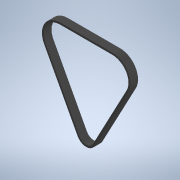
# Autodesk Inventor part: Belt_A
Saved by Autodesk Inventor 2020 (Build 240168000, 168)
## iProperties
Created: 2020-03-07
Part Number: Belt_A
Material: Rubber
Document SubType Name: Modeling
Designer: 10300812
Density: 0.93 g/cm^3
Appearance: Rubber - Black
Mass: 1.6466 g
Surface Area: 29.5089 cm^2
Volume: 1.77053 cm^3
Author: 10300812
Autodesk Inventor part; units mm, degrees
ref_plane "YZ Plane" through (0, 0, 0) normal (1, 0, 0) x (0, 1, 0)
ref_plane "XZ Plane" through (0, 0, 0) normal (0, 1, 0) x (-1, 0, 0)
ref_plane "XY Plane" through (0, 0, 0) normal (0, 0, 1) x (1, 0, 0)
sketch "Sketch1" plane through (0, 0, 0) normal (0, 0, 1) x (1, 0, 0)
  arc A0 (-5.3402, -2.8434) -> (5.3402, -2.8434) centre (0, 0) ccw
  arc A1 (-6.6642, -3.5484) -> (6.6642, -3.5484) centre (0, 0) ccw
  circle A2 centre (-20.5, 52.65) radius 1.25 projected
  circle A3 centre (20.5, 52.65) radius 1.25 projected
  arc A4 (-20.5, 65.35) -> (-31.71, 46.6812) centre (-20.5, 52.65) ccw
  arc A5 (31.71, 46.6812) -> (20.5, 65.35) centre (20.5, 52.65) ccw
  arc A6 (-20.5, 66.85) -> (-33.034, 45.9762) centre (-20.5, 52.65) ccw
  arc A7 (33.034, 45.9762) -> (20.5, 66.85) centre (20.5, 52.65) ccw
  line L0 (-6.6642, -3.5484) -> (-33.034, 45.9762)
  line L1 (-31.71, 46.6812) -> (-5.3402, -2.8434)
  line L2 (6.6642, -3.5484) -> (33.034, 45.9762)
  line L3 (5.3402, -2.8434) -> (31.71, 46.6812)
  line L4 (-20.5, 66.85) -> (20.5, 66.85)
  line L5 (20.5, 65.35) -> (-20.5, 65.35)
  dimension "d0" = 12.1
  dimension "d4" = 25.4
  dimension "d5" = 25.4
  dimension "d6" = 1.5
  dimension "d7" = 1.5
  constraints: 12 end point, 12 point on circle, 8 tangent, 6 centre point, 3 coincident, 3 parallel, 1 horizontal alignment
  measures "d0" diameter of A0
  measures "d4" diameter of A4
  measures "d5" diameter of A5
  measures "d6" radial gap between concentric circles of A4 A6
  measures "d7" radial gap between concentric circles of A5 A7
extrude "Extrusion1" add sketch "Sketch1" along normal blind 6 contours L0 A6 L4 A7 L2 A1
equation "\"d4\" = d5"
body "Solid1"
